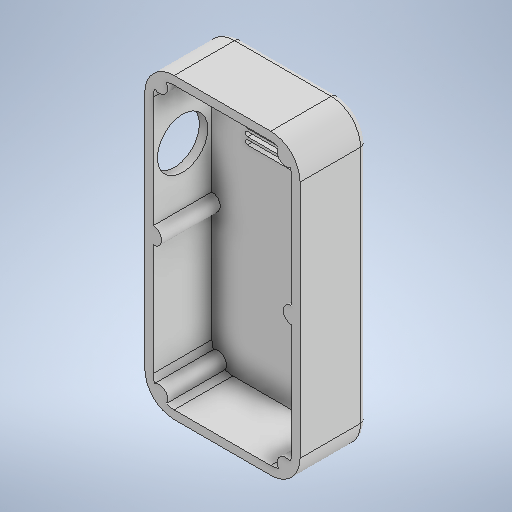
# Autodesk Inventor part: mic-base
Saved by Autodesk Inventor 2025.2 (Build 292293000, 293)
## iProperties
Created: 2025-04-18
Part Number: mic-base
Material: Generic
Document SubType Name: Modeling
Designer: tdeboutte
Density: 1 g/cm^3
Appearance: Default
Author: tdeboutte
Autodesk Inventor part; units mm, degrees
ref_plane "YZ Plane" through (0, 0, 0) normal (1, 0, 0) x (0, 1, 0)
ref_plane "XZ Plane" through (0, 0, 0) normal (0, 1, 0) x (-1, 0, 0)
ref_plane "XY Plane" through (0, 0, 0) normal (0, 0, 1) x (1, 0, 0)
sketch "Sketch1" plane through (0, 0, 0) normal (0, 0, 1) x (1, 0, 0)
  line L0 (7, 0) -> (30, 0)
  line L1 (37, 7) -> (37, 64)
  line L2 (30, 71) -> (7, 71)
  line L3 (0, 64) -> (0, 7)
  arc A0 (7, 71) -> (0, 64) centre (7, 64) ccw
  arc A1 (37, 64) -> (30, 71) centre (30, 64) ccw
  arc A2 (30, 0) -> (37, 7) centre (30, 7) ccw
  arc A3 (0, 7) -> (7, 0) centre (7, 7) ccw
  line L4 (7, 69) -> (30, 69)
  arc A4 (35, 64) -> (30, 69) centre (30, 64) ccw
  line L5 (35, 64) -> (35, 7)
  arc A5 (30, 2) -> (35, 7) centre (30, 7) ccw
  line L6 (30, 2) -> (7, 2)
  arc A6 (2, 7) -> (7, 2) centre (7, 7) ccw
  line L7 (2, 7) -> (2, 64)
  arc A7 (7, 69) -> (2, 64) centre (7, 64) ccw
  point P0 (0, 0)
  point P1 (37, 71)
  point P2 (37, 0)
  point P3 (0, 71)
  dimension "d0" = 37
  dimension "d1" = 71
  dimension "d2" = 7
  dimension "d3" = 2
  constraints: 16 end point, 16 point on circle, 8 centre point, 8 point on line, 8 tangent, 4 parallel, 3 equal radius, 2 perpendicular, 1 horizontal, 7 other
  measures "d0" distance of point (0, 71) point (37, 71)
  measures "d1" distance of point (37, 71) point (37, 0)
  measures "d2" radius of A0
  measures "d3" distance between parallel lines of L2 L4
extrude "Extrusion1" add sketch "Sketch1" along normal blind 14
sketch "Sketch5" plane through (0, 7, 0) normal (-1, 0, 0) x (0, 0, 1)
  line L0 (0, 57) -> (0, 0) projected
  line L1 (0, 0) -> (14, 0) projected
  line L2 (14, 57) -> (14, 0) projected
  line L3 (0, 57) -> (14, 57) projected
  circle A0 centre (7, 44) radius 6
  line L4 (0, 64) -> (14, 64) projected
  point P0 (0, -7)
  point P1 (7, 64)
  dimension "d8" = 12
  dimension "d19" = 20
  constraints: 1 centre point, 1 midpoint
  measures "d8" diameter of A0
  measures "d19" distance of point (7, 64) A0.centre
extrude "Extrusion3" cut sketch "Sketch5" against normal blind 6 contours A0
sketch "Sketch6" plane through (0, 0, 0) normal (0, 0, -1) x (-1, 0, 0)
  arc A0 (-37, 7) -> (-30, 0) centre (-30, 7) ccw projected
  line L0 (-7, 0) -> (-30, 0) projected
  arc A1 (-7, 0) -> (0, 7) centre (-7, 7) ccw projected
  line L1 (0, 64) -> (0, 7) projected
  arc A2 (0, 64) -> (-7, 71) centre (-7, 64) ccw projected
  line L2 (-30, 71) -> (-7, 71) projected
  arc A3 (-30, 71) -> (-37, 64) centre (-30, 64) ccw projected
  line L3 (-37, 7) -> (-37, 64) projected
  line L4 (-2, 7) -> (-2, 64) projected
  arc A4 (-7, 2) -> (-2, 7) centre (-7, 7) ccw projected
  line L5 (-30, 2) -> (-7, 2) projected
  arc A5 (-35, 7) -> (-30, 2) centre (-30, 7) ccw projected
  line L6 (-35, 64) -> (-35, 7) projected
  arc A6 (-30, 69) -> (-35, 64) centre (-30, 64) ccw projected
  line L7 (-7, 69) -> (-30, 69) projected
  arc A7 (-2, 64) -> (-7, 69) centre (-7, 64) ccw projected
  point P0 (0, 0)
extrude "Extrusion4" add sketch "Sketch6" along normal blind 2 contours L3 A3 L2 A2 L1 A1 L0 A0 | A4 L5 A5 L6 A6 L7 A7 L4
fillet "Fillet1" radius 1.6 8 edges at (34.9497, 2.0503, -2) (18.5, 0, -2) (2.0503, 2.0503, -2) (0, 35.5, -2) (2.0503, 68.9497, -2) (18.5, 71, -2) (34.9497, 68.9497, -2) (37, 35.5, -2)
sketch "Sketch7" plane through (0, 0, 0) normal (0, 0, 1) x (1, 0, 0)
  arc A0 (2, 7) -> (7, 2) centre (7, 7) ccw projected
  line L0 (30, 2) -> (7, 2) projected
  arc A1 (30, 2) -> (35, 7) centre (30, 7) ccw projected
  line L1 (35, 64) -> (35, 7) projected
  arc A2 (35, 64) -> (30, 69) centre (30, 64) ccw projected
  line L2 (7, 69) -> (30, 69) projected
  arc A3 (7, 69) -> (2, 64) centre (7, 64) ccw projected
  line L3 (2, 7) -> (2, 64) projected
  line L4 (30, 71) -> (7, 71) projected
  line L5 (18.5, 71) -> (18.5, 0)
  line L6 (7, 0) -> (30, 0) projected
  line L7 (37, 7) -> (37, 64) projected
  line L8 (37, 35.5) -> (0, 35.5)
  line L9 (0, 7) -> (0, 64) projected
  arc A4 (7, 71) -> (0, 64) centre (7, 64) ccw projected
  line L10 (7, 64) -> (14, 64) construction
  circle A5 centre (3.4645, 67.5355) radius 2
  circle A6 centre (33.5355, 67.5355) radius 2
  circle A7 centre (3.4645, 3.4645) radius 2
  circle A8 centre (33.5355, 3.4645) radius 2
  circle A9 centre (2, 35.5) radius 2
  circle A10 centre (35, 35.5) radius 2
  point P0 (0, 0)
  dimension "d15" = 4
  dimension "d16" = 4
  constraints: 6 centre point, 6 end point, 6 midpoint, 3 symmetric about line, 2 horizontal, 2 point on line, 1 point on circle, 1 vertical, 3 other
  measures "d15" diameter of A9
  measures "d16" diameter of A10
extrude "Extrusion5" add sketch "Sketch7" along normal up to surface (14 mm away) contours A7 A0 | A0 A7 | A9 L8 L3 | L3 L8 A9 | L8 A9 L3 | L3 A9 L8 | A5 A3 | A10 L1 L8 | L8 L1 A10 | A3 A5 | L8 A10 L1 | L1 A10 L8 | A8 A1 | A1 A8 | A6 A2 | A2 A6
sketch "Sketch8" plane through (0, 0, 0) normal (0, 0, 1) x (1, 0, 0)
  arc A0 (2, 33.5) -> (2, 37.5) centre (2, 35.5) ccw projected
  line L0 (2, 7) -> (2, 33.5) projected
  arc A1 (2, 7) -> (2.3617, 5.1329) centre (7, 7) ccw projected
  arc A2 (5.1329, 2.3617) -> (2.3617, 5.1329) centre (3.4645, 3.4645) ccw projected
  arc A3 (5.1329, 2.3617) -> (7, 2) centre (7, 7) ccw projected
  line L1 (30, 2) -> (7, 2) projected
  arc A4 (30, 2) -> (31.8671, 2.3617) centre (30, 7) ccw projected
  arc A5 (34.6383, 5.1329) -> (31.8671, 2.3617) centre (33.5355, 3.4645) ccw projected
  arc A6 (34.6383, 5.1329) -> (35, 7) centre (30, 7) ccw projected
  line L2 (35, 33.5) -> (35, 7) projected
  arc A7 (35, 37.5) -> (35, 33.5) centre (35, 35.5) ccw projected
  line L3 (35, 64) -> (35, 37.5) projected
  arc A8 (35, 64) -> (34.6383, 65.8671) centre (30, 64) ccw projected
  arc A9 (31.8671, 68.6383) -> (34.6383, 65.8671) centre (33.5355, 67.5355) ccw projected
  arc A10 (31.8671, 68.6383) -> (30, 69) centre (30, 64) ccw projected
  line L4 (7, 69) -> (30, 69) projected
  arc A11 (7, 69) -> (5.1329, 68.6383) centre (7, 64) ccw projected
  arc A12 (2.3617, 65.8671) -> (5.1329, 68.6383) centre (3.4645, 67.5355) ccw projected
  arc A13 (2.3617, 65.8671) -> (2, 64) centre (7, 64) ccw projected
  line L5 (2, 37.5) -> (2, 64) projected
  line L6 (18.5, 69) -> (18.5, 2)
  line L7 (10.5, 60.45) -> (26.5, 60.45) construction
  line L8 (10.5, 59.9) -> (26.5, 59.9)
  line L9 (26.5, 61) -> (10.5, 61)
  arc A14 (10.5, 61) -> (10.5, 59.9) centre (10.5, 60.45) ccw
  arc A15 (26.5, 59.9) -> (26.5, 61) centre (26.5, 60.45) ccw
  line L10 (18.5, 60.45) -> (34.5, 60.45) construction
  arc A16 (10.5, 59.3) -> (10.5, 58.2) centre (10.5, 58.75) ccw
  line L11 (10.5, 58.2) -> (26.5, 58.2)
  arc A17 (26.5, 58.2) -> (26.5, 59.3) centre (26.5, 58.75) ccw
  line L12 (26.5, 59.3) -> (10.5, 59.3)
  arc A18 (10.5, 57.6) -> (10.5, 56.5) centre (10.5, 57.05) ccw
  line L13 (10.5, 56.5) -> (26.5, 56.5)
  arc A19 (26.5, 56.5) -> (26.5, 57.6) centre (26.5, 57.05) ccw
  line L14 (26.5, 57.6) -> (10.5, 57.6)
  arc A20 (10.5, 55.9) -> (10.5, 54.8) centre (10.5, 55.35) ccw
  line L15 (10.5, 54.8) -> (26.5, 54.8)
  arc A21 (26.5, 54.8) -> (26.5, 55.9) centre (26.5, 55.35) ccw
  line L16 (26.5, 55.9) -> (10.5, 55.9)
  arc A22 (10.5, 54.2) -> (10.5, 53.1) centre (10.5, 53.65) ccw
  line L17 (10.5, 53.1) -> (26.5, 53.1)
  arc A23 (26.5, 53.1) -> (26.5, 54.2) centre (26.5, 53.65) ccw
  line L18 (26.5, 54.2) -> (10.5, 54.2)
  arc A24 (10.5, 52.5) -> (10.5, 51.4) centre (10.5, 51.95) ccw
  line L19 (10.5, 51.4) -> (26.5, 51.4)
  arc A25 (26.5, 51.4) -> (26.5, 52.5) centre (26.5, 51.95) ccw
  line L20 (26.5, 52.5) -> (10.5, 52.5)
  point P0 (0, 0)
  point P1 (18.5, 58.75)
  point P2 (18.5, 57.05)
  point P3 (18.5, 55.35)
  point P4 (18.5, 53.65)
  point P5 (18.5, 51.95)
  point P6 (18.5, 51.4)
  point P7 (18.5, 52.5)
  point P8 (18.5, 54.8)
  point P9 (18.5, 55.9)
  point P10 (18.5, 59.9)
  point P11 (18.5, 61)
  dimension "d20" = 8
  dimension "d22" = 1.1
  dimension "d25" = 1.7
  dimension "d30" = 8
  constraints: 32 end point, 24 point on circle, 12 centre point, 4 tangent, 3 midpoint, 2 vertical, 1 collinear, 1 horizontal, 1 parallel, 1 perpendicular, 1 point on line, 55 other
  measures "d20" distance of L10.start L7.end
  measures "d22" diameter of A15
  measures "d25" distance of L7.start A16.centre
  measures "d30" distance between parallel lines of L4 L9
extrude "Extrusion6" cut sketch "Sketch8" against normal through all contours L19 A24 L20 L6 | L6 L20 A25 L19 | L9 A15 L8 L6 | L6 L8 A14 L9 | L17 A22 L18 L6 | L6 L18 A23 L17 | L12 A17 L11 L6 | L6 L11 A16 L12 | L15 A20 L16 L6 | L6 L16 A21 L15 | L14 A19 L13 L6 | L6 L13 A18 L14
sketch "Sketch9" plane through (0, 0, -2) normal (0, 0, -1) x (-1, 0, 0)
  line L0 (-34.0368, 20.3662) -> (-2.7984, 20.3662) construction
  line L1 (-2.7984, 20.3662) -> (-2.7984, 7.3656) construction
  line L2 (-2.7984, 7.3656) -> (-34.0368, 7.3656) construction
  line L3 (-34.0368, 7.3656) -> (-34.0368, 20.3662) construction
  line L4 (-32.8808, 12.747) -> (-32.8808, 13.9856)
  line L5 (-32.8808, 13.9856) -> (-30.9898, 13.9856)
  spline S0 degree 2 poles (-30.9898, 13.9856) (-30.5852, 13.9856) (-30.1228, 14.5389) (-30.1228, 15.0261) knots 0 0 0 1 2 2 2
  line L6 (-30.1228, 15.0261) -> (-30.1228, 16.5538)
  spline S1 degree 2 poles (-30.1228, 16.5538) (-30.1228, 17.0657) (-30.5852, 17.6272) (-30.9898, 17.6272) knots 0 0 0 1 2 2 2
  line L7 (-30.9898, 17.6272) -> (-32.8808, 17.6272)
  line L8 (-32.8808, 17.6272) -> (-32.8808, 18.8659)
  line L9 (-32.8808, 18.8659) -> (-31.0146, 18.8659)
  spline S2 degree 2 poles (-31.0146, 18.8659) (-30.3127, 18.8659) (-29.3135, 18.3291) (-28.7933, 17.3052) (-28.7933, 16.5785) knots 0 0 0 1 2 3 3 3
  line L10 (-28.7933, 16.5785) -> (-28.7933, 14.9848)
  spline S3 degree 2 poles (-28.7933, 14.9848) (-28.7933, 14.2829) (-29.3218, 13.2755) (-30.321, 12.747) (-31.0146, 12.747) knots 0 0 0 1 2 3 3 3
  line L11 (-31.0146, 12.747) -> (-32.8808, 12.747)
  line L12 (-33.6075, 8.8659) -> (-33.6075, 18.8659)
  line L13 (-33.6075, 18.8659) -> (-32.2946, 18.8659)
  line L14 (-32.2946, 18.8659) -> (-32.2946, 8.8659)
  line L15 (-32.2946, 8.8659) -> (-33.6075, 8.8659)
  spline S4 degree 2 poles (-24.9618, 8.7585) (-25.7462, 8.7585) (-26.861, 9.3531) (-27.4473, 10.4761) (-27.4473, 11.2689) knots 0 0 0 1 2 3 3 3
  line L16 (-27.4473, 11.2689) -> (-27.4473, 16.4629)
  spline S5 degree 2 poles (-27.4473, 16.4629) (-27.4473, 17.2639) (-26.861, 18.387) (-25.7462, 18.9732) (-24.9618, 18.9732) knots 0 0 0 1 2 3 3 3
  spline S6 degree 2 poles (-24.9618, 18.9732) (-24.169, 18.9732) (-23.0625, 18.387) (-22.4762, 17.2639) (-22.4762, 16.4629) knots 0 0 0 1 2 3 3 3
  line L17 (-22.4762, 16.4629) -> (-22.4762, 11.2689)
  spline S7 degree 2 poles (-22.4762, 11.2689) (-22.4762, 10.4761) (-23.0625, 9.3531) (-24.169, 8.7585) (-24.9618, 8.7585) knots 0 0 0 1 2 3 3 3
  spline S8 degree 2 poles (-24.9618, 10.0302) (-24.4085, 10.0302) (-23.7892, 10.6661) (-23.7892, 11.2276) knots 0 0 0 1 2 2 2
  line L18 (-23.7892, 11.2276) -> (-23.7892, 16.5042)
  spline S9 degree 2 poles (-23.7892, 16.5042) (-23.7892, 17.074) (-24.4085, 17.7016) (-24.9618, 17.7016) knots 0 0 0 1 2 2 2
  spline S10 degree 2 poles (-24.9618, 17.7016) (-25.5233, 17.7016) (-26.1344, 17.074) (-26.1344, 16.5042) knots 0 0 0 1 2 2 2
  line L19 (-26.1344, 16.5042) -> (-26.1344, 11.2276)
  spline S11 degree 2 poles (-26.1344, 11.2276) (-26.1344, 10.6661) (-25.5233, 10.0302) (-24.9618, 10.0302) knots 0 0 0 1 2 2 2
  line L20 (-21.1055, 8.8659) -> (-21.1055, 18.8659)
  line L21 (-21.1055, 18.8659) -> (-19.7925, 18.8659)
  line L22 (-19.7925, 18.8659) -> (-19.7925, 8.8659)
  line L23 (-19.7925, 8.8659) -> (-21.1055, 8.8659)
  line L24 (-20.4036, 8.8659) -> (-20.4036, 10.1045)
  line L25 (-20.4036, 10.1045) -> (-16.9519, 10.1045)
  line L26 (-16.9519, 10.1045) -> (-16.9519, 8.8659)
  line L27 (-16.9519, 8.8659) -> (-20.4036, 8.8659)
  line L28 (-14.6232, 18.8659) -> (-14.6232, 8.8659)
  line L29 (-14.6232, 8.8659) -> (-15.9279, 8.8659)
  line L30 (-15.9279, 8.8659) -> (-15.9279, 18.8659)
  line L31 (-15.9279, 18.8659) -> (-14.6232, 18.8659)
  line L32 (-13.2607, 8.8659) -> (-13.2607, 18.8659)
  line L33 (-13.2607, 18.8659) -> (-11.9477, 18.8659)
  line L34 (-11.9477, 18.8659) -> (-11.9477, 8.8659)
  line L35 (-11.9477, 8.8659) -> (-13.2607, 8.8659)
  line L36 (-12.5753, 17.6272) -> (-12.5753, 18.8659)
  line L37 (-12.5753, 18.8659) -> (-8.9667, 18.8659)
  line L38 (-8.9667, 18.8659) -> (-8.9667, 17.6272)
  line L39 (-8.9667, 17.6272) -> (-12.5753, 17.6272)
  line L40 (-12.5753, 8.8659) -> (-12.5753, 10.1045)
  line L41 (-12.5753, 10.1045) -> (-8.9667, 10.1045)
  line L42 (-8.9667, 10.1045) -> (-8.9667, 8.8659)
  line L43 (-8.9667, 8.8659) -> (-12.5753, 8.8659)
  line L44 (-12.5753, 13.2094) -> (-12.5753, 14.4481)
  line L45 (-12.5753, 14.4481) -> (-9.3135, 14.4481)
  line L46 (-9.3135, 14.4481) -> (-9.3135, 13.2094)
  line L47 (-9.3135, 13.2094) -> (-12.5753, 13.2094)
  spline S12 degree 2 poles (-5.5646, 8.7585) (-6.3491, 8.7585) (-7.4391, 9.3035) (-8.0006, 10.3523) (-8.0006, 11.112) knots 0 0 0 1 2 3 3 3
  line L48 (-8.0006, 11.112) -> (-8.0006, 11.6074)
  line L49 (-8.0006, 11.6074) -> (-6.6959, 11.6074)
  line L50 (-6.6959, 11.6074) -> (-6.6959, 11.1615)
  spline S13 degree 2 poles (-6.6959, 11.1615) (-6.6959, 10.6165) (-6.1096, 10.0302) (-5.5646, 10.0302) knots 0 0 0 1 2 2 2
  spline S14 degree 2 poles (-5.5646, 10.0302) (-5.0361, 10.0302) (-4.4746, 10.6165) (-4.4746, 11.1615) knots 0 0 0 1 2 2 2
  line L51 (-4.4746, 11.1615) -> (-4.4746, 12.0368)
  spline S15 degree 2 poles (-4.4746, 12.0368) (-4.4746, 12.4415) (-4.8792, 12.9452) (-5.5233, 13.3002) (-5.8949, 13.4654) knots 0 0 0 1 2 3 3 3
  spline S16 degree 2 poles (-5.8949, 13.4654) (-6.2665, 13.6306) (-7.0014, 14.0352) (-7.6207, 14.605) (-7.9923, 15.4472) (-7.9923, 16.0748) knots 0 0 0 1 2 3 4 4 4
  line L52 (-7.9923, 16.0748) -> (-7.9923, 16.6528)
  spline S17 degree 2 poles (-7.9923, 16.6528) (-7.9923, 17.7759) (-6.7454, 18.9732) (-5.5728, 18.9732) knots 0 0 0 1 2 2 2
  spline S18 degree 2 poles (-5.5728, 18.9732) (-4.4333, 18.9732) (-3.2194, 17.7511) (-3.2194, 16.6281) knots 0 0 0 1 2 2 2
  line L53 (-3.2194, 16.6281) -> (-3.2194, 16.0996)
  line L54 (-3.2194, 16.0996) -> (-4.5241, 16.0996)
  line L55 (-4.5241, 16.0996) -> (-4.5241, 16.5703)
  spline S19 degree 2 poles (-4.5241, 16.5703) (-4.5241, 17.1235) (-5.0609, 17.7016) (-5.5728, 17.7016) knots 0 0 0 1 2 2 2
  spline S20 degree 2 poles (-5.5728, 17.7016) (-6.1178, 17.7016) (-6.6876, 17.1483) (-6.6876, 16.6363) knots 0 0 0 1 2 2 2
  line L56 (-6.6876, 16.6363) -> (-6.6876, 16.017)
  spline S21 degree 2 poles (-6.6876, 16.017) (-6.6876, 15.5711) (-6.25, 15.0426) (-5.5398, 14.6958) (-5.1434, 14.5141) knots 0 0 0 1 2 3 3 3
  spline S22 degree 2 poles (-5.1434, 14.5141) (-4.7966, 14.3572) (-4.103, 14.0021) (-3.5167, 13.4902) (-3.1616, 12.6644) (-3.1616, 12.0286) knots 0 0 0 1 2 3 4 4 4
  line L57 (-3.1616, 12.0286) -> (-3.1616, 11.112)
  spline S23 degree 2 poles (-3.1616, 11.112) (-3.1616, 9.9807) (-4.4003, 8.7585) (-5.5646, 8.7585) knots 0 0 0 1 2 2 2
  point P0 (0, 0)
  constraints: 2 other
extrude "Extrusion7" cut sketch "Sketch9" against normal blind 0.2 contours L11 L14 L15 L12 L13 L8 L7 L5 L4 | L4 L5 L14 L11 | L14 L5 S0 L6 S1 L7 L9 S2 L10 S3 L11 | L7 L8 L9 L14 | S4 L16 S5 S6 L17 S7 | L20 L21 L22 L25 L24 L23 | L24 L25 L22 L23 | L22 L25 L26 L27 | L28 L29 L30 L31 | L32 L33 L36 L39 L34 L45 L44 L47 L41 L40 L35 | L40 L41 L34 L35 | L33 L34 L39 L36 | L34 L41 L42 L43 | L37 L38 L39 L34 | L47 L44 L45 L34 | L34 L45 L46 L47 | S12 L48 L49 L50 S13 S14 L51 S15 S16 L52 S17 S18 L53 L54 L55 S19 S20 L56 S21 S22 L57 S23
body "Solid1"
